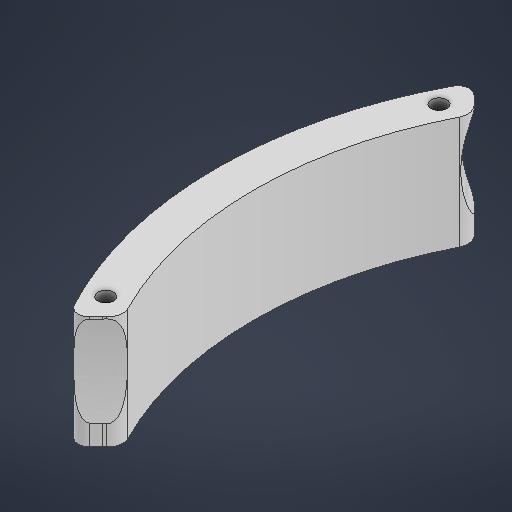
# Autodesk Inventor part: WändeHinten
Saved by Autodesk Inventor 2025.3 (Build 293356000, 356)
## iProperties
Created: 2024-10-20
Part Number: WändeHinten
Material: Generisch
Document SubType Name: Modeling
Designer: Dominik
Density: 1 g/cm^3
Appearance: Vorgabe
Author: Dominik
Autodesk Inventor part; units mm, degrees
ref_plane "YZ Plane" through (0, 0, 0) normal (1, 0, 0) x (0, 1, 0)
ref_plane "XZ Plane" through (0, 0, 0) normal (0, 1, 0) x (-1, 0, 0)
ref_plane "XY Plane" through (0, 0, 0) normal (0, 0, 1) x (1, 0, 0)
sketch "Skizze1" plane through (0, 0, 0) normal (0, 1, 0) x (-1, 0, 0)
  circle A0 centre (-92.6293, 44.3776) radius 1.6
  circle A1 centre (-92.6293, 44.3776) radius 1.6
  circle A2 centre (-92.6293, -44.3776) radius 1.6
  circle A3 centre (-92.6293, -44.3776) radius 1.6
  line L0 (-67.1751, -42.4264) -> (-57.6292, -51.9724)
  arc A4 (-67.1751, -42.4264) -> (-89.6293, -38.3776) centre (-81.3173, -56.5685) ccw
  arc A5 (-89.6293, 38.3776) -> (-89.6293, -38.3776) centre (0, 0) ccw
  arc A6 (-89.6293, 38.3776) -> (-67.1751, 42.4264) centre (-81.3173, 56.5685) ccw
  line L1 (-57.6292, 51.9723) -> (-67.1751, 42.4264)
  line L2 (-57.6292, 51.9723) -> (-26.5165, 20.8596)
  line L3 (-26.5165, 20.8596) -> (-26.5165, -20.8597)
  line L4 (-26.5165, -20.8597) -> (-57.6292, -51.9724)
  line L5 (-51.9723, -57.6292) -> (-20.8596, -26.5165)
  line L6 (-20.8596, -26.5165) -> (20.8597, -26.5165)
  line L7 (20.8597, -26.5165) -> (51.9724, -57.6292)
  line L8 (42.4264, -67.1751) -> (51.9724, -57.6292)
  arc A7 (42.4264, -67.1751) -> (38.3776, -89.6293) centre (56.5685, -81.3173) ccw
  arc A8 (-38.3776, -89.6293) -> (38.3776, -89.6293) centre (0, 0) ccw
  arc A9 (-38.3776, -89.6293) -> (-42.4264, -67.1751) centre (-56.5685, -81.3173) ccw
  line L9 (-51.9723, -57.6292) -> (-42.4264, -67.1751)
  line L10 (57.6292, -51.9723) -> (26.5165, -20.8596)
  line L11 (26.5165, -20.8596) -> (26.5165, 20.8597)
  line L12 (26.5165, 20.8597) -> (57.6292, 51.9724)
  line L13 (67.1751, 42.4264) -> (57.6292, 51.9724)
  arc A10 (67.1751, 42.4264) -> (89.6293, 38.3776) centre (81.3173, 56.5685) ccw
  arc A11 (89.6293, -38.3776) -> (89.6293, 38.3776) centre (0, 0) ccw
  arc A12 (89.6293, -38.3776) -> (67.1751, -42.4264) centre (81.3173, -56.5685) ccw
  line L14 (57.6292, -51.9723) -> (67.1751, -42.4264)
  circle A13 centre (-22.7665, 22.7665) radius 1.6
  circle A14 centre (22.7665, 22.7665) radius 1.6
  circle A15 centre (22.7665, -22.7665) radius 1.6
  circle A16 centre (-22.7665, -22.7665) radius 1.6
  line L15 (-19.0165, 19.0165) -> (19.0165, 19.0165)
  line L16 (19.0165, 19.0165) -> (19.0165, -19.0165)
  line L17 (19.0165, -19.0165) -> (-19.0165, -19.0165)
  line L18 (-19.0165, -19.0165) -> (-19.0165, 19.0165)
  circle A17 centre (-44.3776, -92.6293) radius 1.6
  circle A18 centre (92.6293, 44.3776) radius 1.6
  circle A19 centre (-92.6293, -44.3776) radius 1.6
  circle A20 centre (44.3776, -92.6293) radius 1.6
  circle A21 centre (92.6293, -44.3776) radius 1.6
  circle A22 centre (-92.6293, 44.3776) radius 1.6
  circle A23 centre (45, 91.781) radius 1.6
  circle A24 centre (-45, 91.781) radius 1.6
  arc A25 (12, 71.781) -> (39.8653, 97.0378) centre (12, 99.781) ccw
  line L19 (-12, 71.781) -> (12, 71.781)
  arc A26 (-39.8653, 97.0378) -> (-12, 71.781) centre (-12, 99.781) ccw
  arc A27 (-39.8653, 97.0378) -> (-42.6492, 98.6778) centre (-41.8557, 96.8419) ccw
  arc A28 (-42.6492, 98.6778) -> (-50.5184, 94.8902) centre (0, 0) ccw
  arc A29 (-50.5184, 94.8902) -> (-51.2299, 90.1207) centre (-49.1086, 92.2421) ccw
  line L20 (-49.4975, 88.3883) -> (-51.2299, 90.1207)
  arc A30 (-49.4975, 74.2462) -> (-49.4975, 88.3883) centre (-56.5685, 81.3173) ccw
  line L21 (-74.2462, 49.4975) -> (-49.4975, 74.2462)
  arc A31 (-88.3883, 49.4975) -> (-74.2462, 49.4975) centre (-81.3173, 56.5685) ccw
  line L22 (-90.1208, 51.2299) -> (-88.3883, 49.4975)
  arc A32 (-90.1208, 51.2299) -> (-94.8902, 50.5184) centre (-92.2421, 49.1086) ccw
  arc A33 (-94.8902, 50.5184) -> (-94.8902, -50.5184) centre (0, 0) ccw
  arc A34 (-94.8902, -50.5184) -> (-90.1207, -51.2299) centre (-92.2421, -49.1086) ccw
  line L23 (-88.3883, -49.4975) -> (-90.1207, -51.2299)
  arc A35 (-74.2462, -49.4975) -> (-88.3883, -49.4975) centre (-81.3173, -56.5685) ccw
  line L24 (-49.4975, -74.2462) -> (-74.2462, -49.4975)
  arc A36 (-49.4975, -88.3883) -> (-49.4975, -74.2462) centre (-56.5685, -81.3173) ccw
  line L25 (-51.2299, -90.1208) -> (-49.4975, -88.3883)
  arc A37 (-51.2299, -90.1208) -> (-50.5184, -94.8902) centre (-49.1086, -92.2421) ccw
  arc A38 (-50.5184, -94.8902) -> (50.5184, -94.8902) centre (0, 0) ccw
  arc A39 (50.5184, -94.8902) -> (51.2299, -90.1207) centre (49.1086, -92.2421) ccw
  line L26 (49.4975, -88.3883) -> (51.2299, -90.1207)
  arc A40 (49.4975, -74.2462) -> (49.4975, -88.3883) centre (56.5685, -81.3173) ccw
  line L27 (74.2462, -49.4975) -> (49.4975, -74.2462)
  arc A41 (88.3883, -49.4975) -> (74.2462, -49.4975) centre (81.3173, -56.5685) ccw
  line L28 (90.1208, -51.2299) -> (88.3883, -49.4975)
  arc A42 (90.1208, -51.2299) -> (94.8902, -50.5184) centre (92.2421, -49.1086) ccw
  arc A43 (94.8902, -50.5184) -> (94.8902, 50.5184) centre (0, 0) ccw
  arc A44 (94.8902, 50.5184) -> (90.1207, 51.2299) centre (92.2421, 49.1086) ccw
  line L29 (88.3883, 49.4975) -> (90.1207, 51.2299)
  arc A45 (74.2462, 49.4975) -> (88.3883, 49.4975) centre (81.3173, 56.5685) ccw
  line L30 (49.4975, 74.2462) -> (74.2462, 49.4975)
  arc A46 (49.4975, 88.3883) -> (49.4975, 74.2462) centre (56.5685, 81.3173) ccw
  line L31 (51.2299, 90.1208) -> (49.4975, 88.3883)
  arc A47 (51.2299, 90.1208) -> (50.5184, 94.8902) centre (49.1086, 92.2421) ccw
  arc A48 (50.5184, 94.8902) -> (42.6492, 98.6778) centre (0, 0) ccw
  arc A49 (42.6492, 98.6778) -> (39.8653, 97.0378) centre (41.8557, 96.8419) ccw
  line L32 (51.9723, 57.6292) -> (20.8596, 26.5165)
  line L33 (20.8596, 26.5165) -> (-20.8597, 26.5165)
  line L34 (-20.8597, 26.5165) -> (-51.9724, 57.6292)
  line L35 (-42.4264, 67.1751) -> (-51.9724, 57.6292)
  arc A50 (-42.4264, 67.1751) -> (-38.5642, 72.6085) centre (-56.5685, 81.3173) ccw
  arc A51 (-38.5642, 72.6085) -> (-12, 61.781) centre (-12, 99.781) ccw
  line L36 (12, 61.781) -> (-12, 61.781)
  arc A52 (12, 61.781) -> (38.5642, 72.6085) centre (12, 99.781) ccw
  arc A53 (38.5642, 72.6085) -> (42.4264, 67.1751) centre (56.5685, 81.3173) ccw
  line L37 (51.9723, 57.6292) -> (42.4264, 67.1751)
  circle A54 centre (-48.7904, 67.8822) radius 1.6
  circle A55 centre (48.7904, 67.8823) radius 1.6
  circle A56 centre (67.8822, 48.7904) radius 1.6
  circle A57 centre (-67.8823, 48.7904) radius 1.6
  circle A58 centre (67.8823, -48.7904) radius 1.6
  circle A59 centre (48.7904, -67.8822) radius 1.6
  circle A60 centre (-48.7904, -67.8823) radius 1.6
  circle A61 centre (-67.8822, -48.7904) radius 1.6
  circle A62 centre (0, 0) radius 97.5
  point P0 (85.2233, 47.3629)
  point P1 (89.6293, -38.3776)
  point P2 (85.2233, -47.3629)
  constraints: 76 end point, 76 point on circle, 63 centre point, 3 coincident, 1 concentric
extrude "Extrusion1" add sketch "Skizze1" along normal blind 30 contours A62 A11 A45 L29 A44 A43 A42 L28 A41
fillet "Rundung1" radius 4 2 edges at (-85.2233, 15, 47.3629) (-85.2233, 15, -47.3629)
sketch "Skizze2" plane through (0, 30, 0) normal (0, 1, 0) x (1, 0, 0)
  circle A0 centre (-62.5, -35) radius 1.6
  circle A1 centre (-62.5, 35) radius 1.6
  arc A2 (-89.6293, 38.3776) -> (-67.1751, 42.4264) centre (-81.3173, 56.5685) ccw
  arc A3 (-89.6293, 38.3776) -> (-89.6293, -38.3776) centre (0, 0) ccw
  arc A4 (-67.1751, -42.4264) -> (-89.6293, -38.3776) centre (-81.3173, -56.5685) ccw
  line L0 (-67.1751, -42.4264) -> (-60.4576, -49.1439)
  line L1 (-60.4576, -49.1439) -> (-30, -18.6863)
  line L2 (-30, -18.6863) -> (-30, 18.6863)
  line L3 (-30, 18.6863) -> (-60.4576, 49.1439)
  line L4 (-60.4576, 49.1439) -> (-67.1751, 42.4264)
  point P0 (0, 0)
  point P1 (-26.5912, 40.3648)
  constraints: 10 end point, 6 point on circle, 5 centre point
extrude "Extrusion2" add sketch "Skizze2" along normal blind 3 from surface at -30
sketch "Skizze3" plane through (0, 3, 0) normal (0, 1, 0) x (1, 0, 0)
  circle A0 centre (62.5, -41) radius 1.6
  circle A1 centre (-62.5, -41) radius 1.6
  circle A2 centre (62.5, 41) radius 1.6
  circle A3 centre (-62.5, 41) radius 1.6
  arc A4 (-29.9387, -17.2108) -> (-29.6764, -14.7059) centre (-31.3529, -15.7965) ccw
  arc A5 (-30, -13.6152) -> (-29.6764, -14.7059) centre (-28, -13.6152) ccw
  line L0 (-30, -13.6152) -> (-30, -10.9437)
  arc A6 (-26, -6.9437) -> (-30, -10.9437) centre (-26, -10.9437) ccw
  line L1 (-26, -6.9437) -> (26, -6.9437)
  arc A7 (30, -10.9437) -> (26, -6.9437) centre (26, -10.9437) ccw
  line L2 (30, -10.9437) -> (30, -13.7738)
  arc A8 (29.7071, -14.8159) -> (30, -13.7738) centre (28, -13.7738) ccw
  arc A9 (29.7071, -14.8159) -> (30, -17.2721) centre (31.4142, -15.8579) ccw
  line L3 (30, -17.2721) -> (59.7505, -47.0226)
  arc A10 (59.7505, -47.0226) -> (62.5789, -47.0226) centre (61.1647, -45.6084) ccw
  line L4 (62.5789, -47.0226) -> (62.5789, -47.0226)
  line L5 (62.5789, -47.0226) -> (67.1751, -42.4264)
  arc A11 (89.6293, -38.3776) -> (67.1751, -42.4264) centre (81.3173, -56.5686) ccw
  arc A12 (89.6293, -38.3776) -> (89.6293, 38.3776) centre (0, 0) ccw
  arc A13 (67.1752, 42.4264) -> (89.6293, 38.3776) centre (81.3173, 56.5685) ccw
  line L6 (67.1752, 42.4264) -> (62.5789, 47.0226)
  arc A14 (62.5789, 47.0226) -> (59.7505, 47.0226) centre (61.1647, 45.6084) ccw
  line L7 (59.7505, 47.0226) -> (29.9387, 17.2108)
  arc A15 (29.9387, 17.2108) -> (29.6764, 14.7059) centre (31.3529, 15.7965) ccw
  arc A16 (30, 13.6152) -> (29.6764, 14.7059) centre (28, 13.6152) ccw
  line L8 (30, 13.6152) -> (30, 10.9437)
  arc A17 (26, 6.9437) -> (30, 10.9437) centre (26, 10.9437) ccw
  line L9 (26, 6.9437) -> (-26, 6.9437)
  arc A18 (-30, 10.9437) -> (-26, 6.9437) centre (-26, 10.9437) ccw
  line L10 (-30, 10.9437) -> (-30, 13.7739)
  arc A19 (-29.7071, 14.8158) -> (-30, 13.7739) centre (-28, 13.7739) ccw
  arc A20 (-29.7071, 14.8158) -> (-30, 17.272) centre (-31.4143, 15.8578) ccw
  line L11 (-30, 17.272) -> (-59.7505, 47.0226)
  arc A21 (-59.7505, 47.0226) -> (-62.579, 47.0226) centre (-61.1647, 45.6084) ccw
  line L12 (-62.579, 47.0226) -> (-67.1751, 42.4264)
  arc A22 (-89.6293, 38.3776) -> (-67.1751, 42.4264) centre (-81.3173, 56.5685) ccw
  arc A23 (-89.6293, 38.3776) -> (-89.6293, -38.3776) centre (0, 0) ccw
  arc A24 (-67.1751, -42.4264) -> (-89.6293, -38.3776) centre (-81.3173, -56.5685) ccw
  line L13 (-67.1751, -42.4264) -> (-62.5789, -47.0226)
  arc A25 (-62.5789, -47.0226) -> (-59.7505, -47.0226) centre (-61.1647, -45.6084) ccw
  line L14 (-59.7505, -47.0226) -> (-29.9387, -17.2108)
  point P0 (0, 0)
  point P1 (0, 0)
  constraints: 44 point on circle, 30 end point, 26 centre point
extrude "Extrusion3" cut sketch "Skizze3" against normal blind 10 contours A1 | A3
sketch "Skizze4" plane through (0, 3, 0) normal (0, 1, 0) x (1, 0, 0)
  line L0 (-64.6409, 43.0746) -> (-60.307, 43.0746)
  line L1 (-60.307, 43.0746) -> (-60.307, -43.3308)
  line L2 (-60.307, -43.3308) -> (-64.6409, -43.3308)
  line L3 (-64.6409, -43.3308) -> (-64.6409, 43.0746)
  line L4 (-64.6409, 37.5016) -> (-60.307, 37.5016)
  line L5 (-60.307, 37.5016) -> (-60.307, -37.9108)
  line L6 (-60.307, -37.9108) -> (-64.6409, -37.9108)
  line L7 (-64.6409, -37.9108) -> (-64.6409, 37.5016)
  point P0 (0, 0)
  constraints: 16 end point, 4 parallel, 2 horizontal, 2 perpendicular, 2 point on line
extrude "Extrusion4" add sketch "Skizze4" against normal blind 3 contours L4 L1 L6 L3
sketch "Skizze6" plane through (0, 3, 0) normal (0, 1, 0) x (1, 0, 0)
  circle A0 centre (-62.5, 41) radius 1.6
  circle A1 centre (-62.5, 41) radius 6.2
  circle A2 centre (-62.5, -41) radius 1.6
  circle A3 centre (-62.5, -41) radius 6.2
  circle A4 centre (-62.5, -41) radius 2.1
  line L0 (-60.4576, -49.1439) -> (-67.1751, -42.4264) projected
  arc A5 (-62.4023, -47.1992) -> (-68.7, -41) centre (-263.9524, -245.6516) ccw
  circle A6 centre (-62.5, 41) radius 2.1
  arc A7 (-68.7, 41) -> (-62.5, 47.2) centre (-163.1895, 141.6895) ccw
  line L1 (-67.1751, 42.4264) -> (-60.4576, 49.1439) projected
  point P0 (0, 0)
  point P1 (-62.4023, 47.1992)
  point P2 (-65.5508, 44.0508)
  dimension "d14" = 12.4
  dimension "d15" = 12.4
  dimension "d18" = 4.2
  dimension "d19" = 4.2
  constraints: 8 centre point, 8 point on circle, 6 coincident, 1 point on line, 1 tangent
  measures "d14" diameter of A1
  measures "d15" diameter of A3
  measures "d18" diameter of A4
  measures "d19" diameter of A6
extrude "Extrusion6" add sketch "Skizze6" along normal blind 22 contours A7 L1 A1 | A3 A5 picked at (-63.7326, 44.7378)
fillet "Rundung2" radius 4 4 edges at (-62.4023, 14, 47.1992) (-68.7, 14, 41) (-62.4023, 14, -47.1992) (-68.7, 14, -41)
fillet "Rundung3" radius 4 1 edges at (-30, 1.5, 18.6863)
fillet "Rundung4" radius 4 1 edges at (-30, 1.5, -18.6863)
fillet "Rundung5" radius 4 1 edges at (-60.4576, 1.5, -49.1439)
fillet "Rundung6" radius 4 1 edges at (-89.6293, 1.5, -38.3776)
fillet "Rundung7" radius 4 2 edges at (-89.6293, 1.5, 38.3776) (-60.4576, 1.5, 49.1439)
sketch "Skizze7" plane through (0, 30, 0) normal (0, 1, 0) x (1, 0, 0)
  line L0 (0, 0) -> (0, -29.0841) construction
  line L1 (0, 0) -> (-84.8528, -84.8528)
  line L2 (-68.9429, -111.3693) -> (-111.3693, -68.9429)
  line L3 (-111.3693, -68.9429) -> (-100.7627, -58.3363)
  line L4 (-100.7627, -58.3363) -> (-58.3363, -100.7627)
  line L5 (-58.3363, -100.7627) -> (-68.9429, -111.3693)
  line L6 (-68.9429, -111.3693) -> (-100.7627, -58.3363) construction
  line L7 (-111.3693, -68.9429) -> (-58.3363, -100.7627) construction
  dimension "d29" = 45
  dimension "d30" = 120
  dimension "d31" = 60
  dimension "d32" = 15
  constraints: 16 end point, 2 midpoint, 2 parallel, 1 perpendicular, 1 vertical
  measures "d29" angle of L1 L0
  measures "d30" distance of L0.start L1.end
  measures "d31" distance of L2.start L2.end
  measures "d32" distance of L2.end L3.end
extrude "Extrusion7" add sketch "Skizze7" against normal up to surface (30 mm away)
sketch "Skizze8" plane through (-68.9429, 0, 111.3693) normal (-0.7071068, 0, 0.7071068) x (0.7071068, 0, 0.7071068)
  line L0 (-30, 0) -> (-30, 17.5)
  circle A0 centre (-30, 17.5) radius 30
  line L1 (0, 30) -> (-60, 30) projected
  line L2 (0, 30) -> (0, 0) projected
  line L3 (-60, 30) -> (0, 30)
  line L4 (0, 30) -> (0, 0)
  line L5 (0, 0) -> (-60, 0)
  line L6 (-60, 0) -> (-60, 30)
  point P0 (-60, 17.5)
  point P1 (-54.367, 0)
  point P2 (-57.2718, 30)
  point P3 (-5.633, 0)
  point P4 (-2.7282, 30)
  point P5 (0, 17.5)
  dimension "d35" = 17.5
  dimension "d36" = 60
  constraints: 10 end point, 2 parallel, 1 centre point, 1 coincident, 1 horizontal, 1 perpendicular, 1 vertical
  measures "d35" distance of L0.start L0.end
  measures "d36" diameter of A0
extrude "Extrusion8" cut sketch "Skizze8" against normal up to surface (15 mm away) contours A0 L5 L1 | L2 L5 A0 | A0 L1 L2 | A0 L6 L1 | L5 L6 A0
extrude "Extrusion9" cut sketch "Skizze8" against normal blind 45 contours A0 L5 L1 | L1 A0 | A0 L5
mirror "Spiegeln1" about plane through (0, 0, 0) normal (0, 0, 1) of "Extrusion9", "Extrusion8"
sketch "Skizze9" plane through (-30, 3, 17.0294) normal (0, 1, 0) x (1, 0, 0)
  circle A0 centre (30, 17.0294) radius 97.5
  constraints: 1 centre point, 1 coincident
extrude "Extrusion10" cut sketch "Skizze9" along normal mid plane 100
sketch "Skizze10" plane through (0, 30, 0) normal (0, 1, 0) x (1, 0, 0)
  circle A0 centre (-92.6293, 44.3776) radius 1.6 projected
  circle A1 centre (-92.6293, 44.3776) radius 2.1
  circle A2 centre (-92.6293, -44.3776) radius 1.6 projected
  circle A3 centre (-92.6293, -44.3776) radius 2.1
  point P0 (0, 0)
  dimension "d43" = 4.2
  dimension "d44" = 4.2
  constraints: 2 centre point, 2 coincident
  measures "d43" diameter of A1
  measures "d44" diameter of A3
extrude "Extrusion11" cut sketch "Skizze10" against normal up to surface (30 mm away) contours A0 | A1 | A2 | A3
